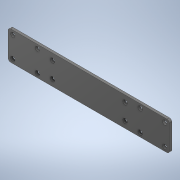
# Autodesk Inventor part: de ga con truot
Saved by Autodesk Inventor 2020 (Build 240168000, 168)
## iProperties
Created: 2021-05-31
Part Number: de ga con truot
Material: Generic
Document SubType Name: Modeling
Designer: Admin
Density: 1 g/cm^3
Appearance: Smooth - Black
Author: Admin
Autodesk Inventor part; units mm, degrees
ref_plane "YZ Plane" through (0, 0, 0) normal (1, 0, 0) x (0, 1, 0)
ref_plane "XZ Plane" through (0, 0, 0) normal (0, 1, 0) x (-1, 0, 0)
ref_plane "XY Plane" through (0, 0, 0) normal (0, 0, 1) x (1, 0, 0)
sketch "Sketch1" plane through (0, 0, 0) normal (0, 0, 1) x (1, 0, 0)
  line L0 (-100, -18) -> (100, -18)
  line L1 (100, -18) -> (100, 18)
  line L2 (100, 18) -> (-100, 18)
  line L3 (-100, 18) -> (-100, -18)
  line L4 (-100, -18) -> (100, 18) construction
  line L5 (100, -18) -> (-100, 18) construction
  point P0 (0, 0)
  dimension "d0" = 200
  dimension "d1" = 36
  constraints: 12 end point, 2 midpoint, 2 parallel, 1 horizontal, 1 perpendicular
  measures "d0" distance of L2.end L1.end
  measures "d1" distance of L1.end L0.end
extrude "Extrusion1" add sketch "Sketch1" along normal blind 3
sketch "Sketch2" plane through (0, 0, 3) normal (0, 0, 1) x (1, 0, 0)
  line L0 (-94.25, -13) -> (-63.75, -13)
  line L1 (-63.75, -13) -> (-63.75, 13)
  line L2 (-63.75, 13) -> (-94.25, 13)
  line L3 (-94.25, 13) -> (-94.25, -13)
  line L4 (-94.25, -13) -> (-63.75, 13) construction
  line L5 (-63.75, -13) -> (-94.25, 13) construction
  line L6 (100, 18) -> (-100, 18) projected
  line L7 (-100, -18) -> (-58, -18)
  line L8 (-58, -18) -> (-58, 18)
  line L9 (-58, 18) -> (-100, 18)
  line L10 (-100, 18) -> (-100, -18)
  line L11 (-100, -18) -> (-58, 18) construction
  line L12 (-58, -18) -> (-100, 18) construction
  line L13 (-100, 18) -> (-100, -18) projected
  circle A0 centre (-94.25, 13) radius 2.75
  circle A1 centre (-63.75, 13) radius 2.75
  circle A2 centre (-94.25, -13) radius 2.75
  circle A3 centre (-63.75, -13) radius 2.75
  line L14 (63.75, -13) -> (94.25, -13)
  line L15 (94.25, -13) -> (94.25, 13)
  line L16 (94.25, 13) -> (63.75, 13)
  line L17 (63.75, 13) -> (63.75, -13)
  line L18 (63.75, -13) -> (94.25, 13) construction
  line L19 (94.25, -13) -> (63.75, 13) construction
  line L20 (58, -18) -> (100, -18)
  line L21 (100, -18) -> (100, 18)
  line L22 (100, 18) -> (58, 18)
  line L23 (58, 18) -> (58, -18)
  line L24 (58, -18) -> (100, 18) construction
  line L25 (100, -18) -> (58, 18) construction
  circle A4 centre (63.75, 13) radius 2.75
  circle A5 centre (94.25, 13) radius 2.75
  circle A6 centre (63.75, -13) radius 2.75
  circle A7 centre (94.25, -13) radius 2.75
  line L26 (100, -18) -> (100, 18) projected
  point P0 (0, 0)
  point P1 (-79, 0)
  point P2 (-79, 0)
  point P3 (79, 0)
  point P4 (79, 0)
  dimension "d4" = 30.5
  dimension "d5" = 26
  dimension "d6" = 42
  dimension "d7" = 0
  dimension "d8" = 0
  dimension "d9" = 5.5
  dimension "d10" = 5.5
  dimension "d11" = 5.5
  dimension "d12" = 5.5
  dimension "d13" = 30.5
  dimension "d14" = 26
  dimension "d15" = 42
  dimension "d16" = 0
  dimension "d17" = 5.5
  dimension "d18" = 5.5
  dimension "d19" = 5.5
  dimension "d20" = 5.5
  dimension "d21" = 0
  dimension "d22" = 36
  constraints: 48 end point, 8 centre point, 8 coincident, 8 midpoint, 8 parallel, 4 horizontal, 4 perpendicular, 1 point on line
  measures "d4" distance of L2.end L1.end
  measures "d5" distance of L1.end L0.end
  measures "d6" distance of L9.end L8.end
  measures "d7" distance between parallel lines of L13 L10
  measures "d8" distance of point (-79, 0) point (-79, 0)
  measures "d9" diameter of A0
  measures "d10" diameter of A1
  measures "d11" diameter of A2
  measures "d12" diameter of A3
  measures "d13" distance of L16.end L16.start
  measures "d14" distance of L16.start L15.start
  measures "d15" distance of L22.end L22.start
  measures "d16" distance of point (79, 0) point (79, 0)
  measures "d17" diameter of A4
  measures "d18" diameter of A5
  measures "d19" diameter of A6
  measures "d20" diameter of A7
  measures "d21" distance between parallel lines of L21 L26
  measures "d22" distance between parallel lines of L20 L6
extrude "Extrusion2" cut sketch "Sketch2" against normal blind 3 contours L3 A2 L0 | L0 A2 L3 | A3 L1 L0 | L0 L1 A3 | A0 L2 L3 | L3 L2 A0 | A1 L2 L1 | L1 L2 A1 | L17 A6 L14 | L14 A6 L17 | A7 L15 L14 | L14 L15 A7 | A4 L16 L17 | L17 L16 A4 | A5 L16 L15 | L15 L16 A5
fillet "Fillet1" radius 3 4 edges at (100, 18, 1.5) (100, -18, 1.5) (-100, -18, 1.5) (-100, 18, 1.5)
sketch "Sketch3" plane through (0, 0, 3) normal (0, 0, 1) x (1, 0, 0)
  line L0 (-45, -10) -> (45, -10)
  line L1 (45, -10) -> (45, 10)
  line L2 (45, 10) -> (-45, 10)
  line L3 (-45, 10) -> (-45, -10)
  line L4 (-45, -10) -> (45, 10) construction
  line L5 (45, -10) -> (-45, 10) construction
  point P0 (0, 0)
  dimension "d26" = 90
  dimension "d27" = 20
  constraints: 12 end point, 2 midpoint, 2 parallel, 1 horizontal, 1 perpendicular
  measures "d26" distance of L2.end L1.end
  measures "d27" distance of L1.end L0.end
hole "Hole1" at (-45, 10, 3) at (45, 10, 3) at (45, -10, 3) at (-45, -10, 3) direction (0, 0, -1) diameter 5.5 end through all
body "Solid1"
